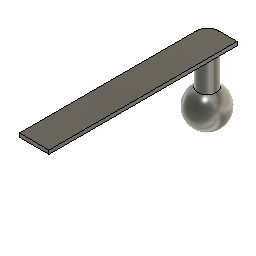
plastic model 1 (Autodesk Fusion 360 design; units mm, degrees)
Autodesk Fusion 360 part; units mm, degrees
sphere "SpherePrimitive1" add diameter 100 placed x (1, 0, 0) y (0, 0, -1) z (0, 1, 0) at (0, 0, 0)
sketch "Sketch2" plane through (0, 0, 0) normal (0, 0, 1) x (1, 0, 0)
  circle A0 centre (0, 0) radius 25
  dimension "d2" = 50
  constraint coincident A0.centre origin
  measures "d2" diameter of A0
extrude "Extrude1" cut sketch "Sketch2" along normal blind 90
extrude "Extrude2" add 1 faces at (-6.7759, -1.242, 0) along direction (0, 0, 1) blind 150
sketch "Sketch3" plane through (0, 0, 0) normal (0, 0, 1) x (1, 0, 0)
box "BoxPrimitive1" cut length 35 width 33.501 height 205 placed x (0, -1, 0) y (1, 0, 0) z (0, 0, 1) at (-16.9474, 18.4254, 0)
extrude "Extrude3" add 1 faces at (-5.7804, -4.9079, 0) along direction (0, 0, 1) blind 220
extrude "Extrude4" cut 1 faces at (-5.7804, -4.9079, 220) along direction (0, 0, -1) blind 60
extrude "Extrude5" add 1 faces at (-5.7804, -16.5746, 156.6667) along direction (0, -1, 0) blind 400
extrude "Extrude6" add 1 faces at (-5.7636, 18.4254, 156.6667) along direction (0, 1, 0) blind 10
extrude "Extrude7" add 1 faces at (-16.9474, -135.5094, 156.6667) along direction (-1, 0, 0) blind 10
extrude "Extrude8" add 1 faces at (16.5536, -135.6279, 156.6667) along direction (1, 0, 0) blind 10
fillet "Fillet1" radius 30 1 edges at (-26.9474, 28.4254, 101.6408)
extrude "Extrude9" add 1 faces at (26.5536, -268.2413, 153.3333) along direction (1, 0, 0) blind 25
extrude "Extrude10" add 1 faces at (-0.7804, -416.5746, 153.3333) along direction (0, -1, 0) blind 50
extrude "Extrude11" add 1 faces at (-0.7804, -466.5746, 153.3333) along direction (0, -1, 0) blind 5
